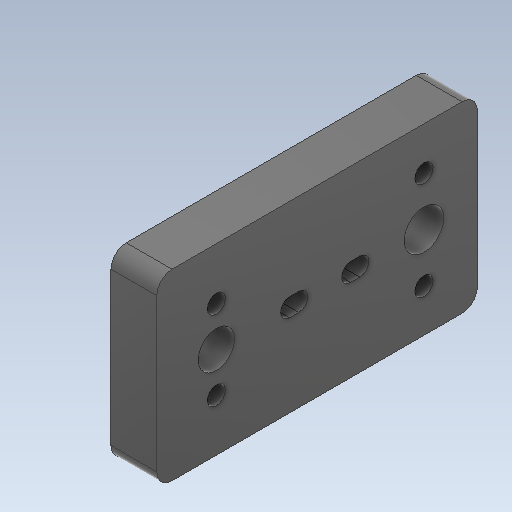
# Autodesk Inventor part: 0008-10-033
Saved by Autodesk Inventor 2020 (Build 240168000, 168)
## iProperties
Created: 2021-03-06
Part Number: 0008-10-033
Material: ABS Plastic
Document SubType Name: Modeling
Designer: Iulian Bors
Density: 1.06 g/cm^3
Appearance: Smooth - White
Mass: 108.095 g
Surface Area: 226.81 cm^2
Volume: 101.976 cm^3
Description: Suport Axa Z
Author: Iulian Bors
Subject: 033
Autodesk Inventor part; units mm, degrees
ref_plane "YZ Plane" through (0, 0, 0) normal (1, 0, 0) x (0, 1, 0)
ref_plane "XZ Plane" through (0, 0, 0) normal (0, 1, 0) x (-1, 0, 0)
ref_plane "XY Plane" through (0, 0, 0) normal (0, 0, 1) x (1, 0, 0)
sketch "Sketch1" plane through (0, 0, 0) normal (0, 0, 1) x (1, 0, 0)
  line L0 (-40, 7.5) -> (0, 7.5)
  line L1 (0, 7.5) -> (0, -7.5)
  line L2 (0, -7.5) -> (-40, -7.5)
  line L3 (-40, -7.5) -> (-40, 7.5)
  line L4 (-15, 52.5) -> (0, 52.5)
  line L5 (0, 52.5) -> (0, 7.5)
  line L6 (0, 7.5) -> (-15, 7.5)
  line L7 (-15, 7.5) -> (-15, 52.5)
  point P0 (0, 0)
  point P1 (-15, 7.5)
  dimension "d0" = 15
  dimension "d1" = 40
  dimension "d2" = 60
  constraints: 16 end point, 4 parallel, 3 perpendicular, 2 horizontal, 1 collinear, 1 midpoint, 1 point on line
  measures "d0" distance of L2.end L0.start
  measures "d1" distance of L1.end L2.end
  measures "d2" distance between parallel lines of L2 L4
extrude "Extrusion1" add sketch "Sketch1" along normal blind 40
sketch "Sketch2" plane through (-15, 7.5, 0) normal (-1, 0, 0) x (0, 0, 1)
  line L0 (8.5, 15) -> (11.5, 15) construction
  line L1 (8.5, 12) -> (11.5, 12)
  line L2 (11.5, 18) -> (8.5, 18)
  arc A0 (8.5, 18) -> (8.5, 12) centre (8.5, 15) ccw
  arc A1 (11.5, 12) -> (11.5, 18) centre (11.5, 15) ccw
  line L3 (0, 45) -> (0, 0) projected
  line L4 (0, 45) -> (40, 45) projected
  line L5 (20, 21.547) -> (20, 15) construction
  line L6 (31.5, 15) -> (28.5, 15) construction
  line L7 (31.5, 12) -> (28.5, 12)
  line L8 (28.5, 18) -> (31.5, 18)
  arc A2 (31.5, 12) -> (31.5, 18) centre (31.5, 15) ccw
  arc A3 (28.5, 18) -> (28.5, 12) centre (28.5, 15) ccw
  point P0 (0, -7.5)
  point P1 (10, 15)
  point P2 (20, 18.2735)
  point P3 (20, 45)
  point P4 (30, 15)
  dimension "d5" = 6
  dimension "d6" = 3
  dimension "d7" = 10
  dimension "d8" = 30
  constraints: 18 end point, 8 point on circle, 7 symmetric about line, 4 centre point, 4 tangent, 3 midpoint, 1 horizontal, 1 parallel, 1 vertical, 1 vertical alignment, 2 other
  measures "d5" diameter of A1
  measures "d6" distance of L0.start L0.end
  measures "d7" distance from line of L3 point (10, 15)
  measures "d8" distance between parallel lines of L0 L4
extrude "Extrusion2" cut sketch "Sketch2" against normal through all
sketch "Sketch3" plane through (-40, 7.5, 0) normal (0, 1, 0) x (1, 0, 0)
  line L0 (10, -8.5) -> (10, -11.5) construction
  line L1 (7, -8.5) -> (7, -11.5)
  line L2 (13, -11.5) -> (13, -8.5)
  arc A0 (13, -8.5) -> (7, -8.5) centre (10, -8.5) ccw
  arc A1 (7, -11.5) -> (13, -11.5) centre (10, -11.5) ccw
  line L3 (25, 0) -> (0, 0) projected
  line L4 (0, 0) -> (0, -40) projected
  line L5 (15.2557, -20) -> (9.287, -20) construction
  line L6 (10, -31.5) -> (10, -28.5) construction
  line L7 (7, -31.5) -> (7, -28.5)
  line L8 (13, -28.5) -> (13, -31.5)
  arc A2 (7, -31.5) -> (13, -31.5) centre (10, -31.5) ccw
  arc A3 (13, -28.5) -> (7, -28.5) centre (10, -28.5) ccw
  point P0 (40, 0)
  point P1 (10, -10)
  point P2 (12.2713, -20)
  point P3 (0, -20)
  point P4 (10, -30)
  dimension "d11" = 3
  dimension "d12" = 6
  dimension "d13" = 10
  dimension "d14" = 10
  constraints: 18 end point, 8 point on circle, 7 symmetric about line, 4 centre point, 4 tangent, 3 midpoint, 1 horizontal, 1 horizontal alignment, 1 parallel, 1 vertical, 2 other
  measures "d11" distance of L0.start L0.end
  measures "d12" distance between parallel lines of L1 L2
  measures "d13" distance from line of L3 point (10, -10)
  measures "d14" distance between parallel lines of L4 L0
extrude "Extrusion3" cut sketch "Sketch3" against normal through all
sketch "Sketch5" plane through (0, 0, 0) normal (0, 0, -1) x (-1, 0, 0)
  line L0 (0, -7.5) -> (15, -7.5)
  line L1 (15, -7.5) -> (15, 52.5)
  line L2 (15, 52.5) -> (0, 52.5)
  line L3 (0, 52.5) -> (0, -7.5)
  line L4 (0, -7.5) -> (0, 52.5) projected
  line L5 (40, -7.5) -> (0, -7.5) projected
  line L6 (0, 52.5) -> (15, 52.5) projected
  line L7 (15, 52.5) -> (15, 7.5) projected
  point P0 (0, 0)
  point P1 (10, 15)
  constraints: 8 end point, 3 collinear, 2 parallel, 1 horizontal, 1 perpendicular, 1 vertical, 1 other
extrude "Extrusion4" add sketch "Sketch5" along normal blind 30
sketch "Sketch6" plane through (0, -7.5, 40) normal (1, 0, 0) x (0, 0, -1)
  circle A0 centre (52.5, 14) radius 3
  circle A1 centre (52.5, 46) radius 3
  line L0 (70, 0) -> (0, 0) projected
  line L1 (70, 60) -> (70, 0) projected
  circle A2 centre (52.5, 30) radius 6.5
  point P0 (40, 7.5)
  dimension "d23" = 32
  dimension "d24" = 14
  dimension "d25" = 17.5
  dimension "d26" = 6
  dimension "d31" = 13
  dimension "d32" = 16
  constraints: 3 centre point, 2 vertical alignment, 1 equal radius
  measures "d23" distance of A1.centre A0.centre
  measures "d24" distance from line of L0 A0.centre
  measures "d25" distance from line of A0.centre L1
  measures "d26" diameter of A0
  measures "d31" diameter of A2
  measures "d32" distance of A2.centre A0.centre
extrude "Extrusion5" cut sketch "Sketch6" against normal through all
sketch "Sketch7" plane through (0, 0, 40) normal (0, 0, 1) x (1, 0, 0)
  line L0 (0, 52.5) -> (-15, 52.5)
  line L1 (-15, 52.5) -> (-15, -7.5)
  line L2 (-15, -7.5) -> (0, -7.5)
  line L3 (0, -7.5) -> (0, 52.5)
  line L4 (0, -7.5) -> (0, 52.5) projected
  line L5 (0, 52.5) -> (-15, 52.5) projected
  line L6 (-15, 52.5) -> (-15, 7.5) projected
  line L7 (-40, -7.5) -> (0, -7.5) projected
  point P0 (0, 0)
  point P1 (-10, 15)
  constraints: 8 end point, 3 collinear, 2 parallel, 1 horizontal, 1 perpendicular, 1 vertical, 1 other
extrude "Extrusion6" add sketch "Sketch7" along normal blind 35
sketch "Sketch8" plane through (0, -7.5, -30) normal (1, 0, 0) x (0, 0, -1)
  circle A0 centre (-85.5, 30) radius 6
  circle A1 centre (-85.5, 17) radius 3
  circle A2 centre (-85.5, 43) radius 3
  line L0 (-105, 60) -> (0, 60) projected
  line L1 (-105, 0) -> (-105, 60) projected
  point P0 (-30, 7.5)
  dimension "d33" = 12
  dimension "d34" = 6
  dimension "d35" = 17
  dimension "d36" = 19.5
  dimension "d37" = 26
  dimension "d38" = 13
  constraints: 3 centre point, 2 vertical alignment, 1 equal radius
  measures "d33" diameter of A0
  measures "d34" diameter of A2
  measures "d35" distance from line of A2.centre L0
  measures "d36" distance from line of A2.centre L1
  measures "d37" distance of A1.centre A2.centre
  measures "d38" distance of A0.centre A2.centre
extrude "Extrusion7" cut sketch "Sketch8" against normal through all
chamfer "Chamfer2" distance 5 angle 45 3 edges at (-15, 0, 40) (-15, 7.5, 20) (-15, 0, 0)
fillet "Fillet2" radius 5 4 edges at (-7.5, 52.5, 75) (-7.5, -7.5, 75) (-7.5, 52.5, -30) (-7.5, -7.5, -30)
equation "\"d32\" = 0.5 * d23"
equation "\"d38\" = 0.5 * d37"
body "Solid1"
